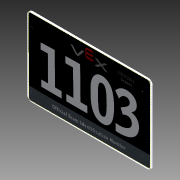
# Autodesk Inventor part: 1103 ID Plate
Saved by Autodesk Inventor 2012 (Build 160160000, 160)
## iProperties
Created: 2011-09-16
Part Number: 1103 ID Plate
Material: Default
Document SubType Name: Modeling
Designer: Wade
Density: 1 g/cm^3
Author: Wade
Autodesk Inventor part; units mm, degrees
ref_plane "YZ Plane" through (0, 0, 0) normal (1, 0, 0) x (0, 1, 0)
ref_plane "XZ Plane" through (0, 0, 0) normal (0, 1, 0) x (-1, 0, 0)
sketch "Sketch1" plane through (0, 0, 0) normal (0, 0, 1) x (1, 0, 0)
  line L0 (0, 0) -> (85.725, 0)
  line L1 (85.725, 0) -> (85.725, -53.975)
  line L2 (85.725, -53.975) -> (0, -53.975)
  line L3 (0, -53.975) -> (0, 0)
  line L4 (0, 0) -> (4.7625, 0)
  line L5 (0, -7.9375) -> (0, 0)
  line L6 (0, -53.975) -> (4.7625, -53.975)
  line L7 (0, -46.0375) -> (0, -53.975)
  line L8 (85.725, 0) -> (80.9625, 0)
  line L9 (85.725, -7.9375) -> (85.725, 0)
  line L10 (85.725, -53.975) -> (80.9625, -53.975)
  line L11 (85.725, -46.0375) -> (85.725, -53.975)
  circle A0 centre (80.9625, -46.0375) radius 2.3114
  circle A1 centre (80.9625, -7.9375) radius 2.3114
  circle A2 centre (4.7625, -7.9375) radius 2.3114
  circle A3 centre (4.7625, -46.0375) radius 2.3114
  dimension "d0" = 85.725
  dimension "d1" = 53.975
  dimension "d10" = 4.6228
  dimension "d11" = 4.6228
  dimension "d12" = 4.6228
  dimension "d13" = 4.6228
  constraints: 24 end point, 5 horizontal, 4 centre point, 2 parallel, 1 perpendicular
  measures "d0" distance of L1.end L2.end
  measures "d1" distance of L0.end L1.end
  measures "d10" diameter of A0
  measures "d11" diameter of A1
  measures "d12" diameter of A2
  measures "d13" diameter of A3
extrude "Extrusion2" add sketch "Sketch1" along normal blind 0.7937
fillet "Fillet1" radius 3.175 4 edges at (0, 0, 0.3969) (0, -53.975, 0.3969) (85.725, 0, 0.3969) (85.725, -53.975, 0.3969)
ref_plane "Work Plane2" through (1.5748, -52.4002, 1.0732) normal (0, 0, 1) x (1, 0, 0)
sketch "Sketch12" plane through (0, 0, 0.7937) normal (0, 0, 1) x (1, 0, 0)
  line L0 (0.9299, -0.9299) -> (84.6106, -0.6351) construction
  line L1 (84.6106, -0.6351) -> (84.7953, -53.0451) construction
  line L2 (84.7953, -53.0451) -> (1.1146, -53.3399) construction
  line L3 (1.1146, -53.3399) -> (0.9299, -0.9299) construction
  constraints: 2 other
body "Solid2"
